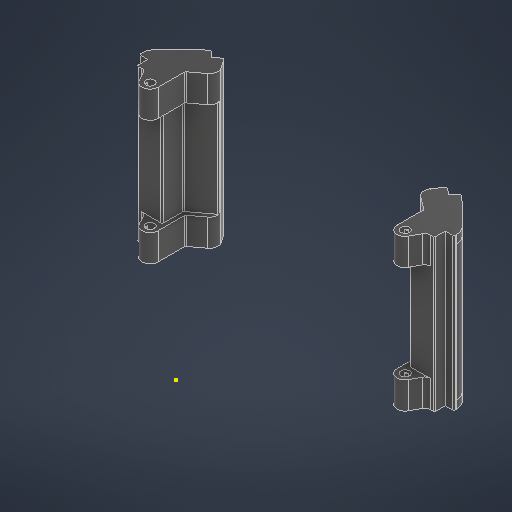
# Autodesk Inventor part: Esquinero Trasero
Saved by Autodesk Inventor 2026.2 (Build 302298000, 298)
## iProperties
Created: 2025-03-12
Part Number: Esquinero Trasero
Material: Generic
Document SubType Name: Modeling
Designer: cdavi
Density: 1 g/cm^3
Appearance: Dark Gray
Author: cdavi
Autodesk Inventor part; units mm, degrees
ref_plane "YZ Plane" through (0, 0, 0) normal (1, 0, 0) x (0, 1, 0)
ref_plane "XZ Plane" through (0, 0, 0) normal (0, 1, 0) x (-1, 0, 0)
ref_plane "XY Plane" through (0, 0, 0) normal (0, 0, 1) x (1, 0, 0)
sketch "Sketch1" plane through (0, 0, 0) normal (0, 1, 0) x (-1, 0, 0)
  line L0 (50.9902, 55) -> (-50.9902, 55)
  line L1 (12, -62.25) -> (-12, -62.25)
  line L2 (-12, -60) -> (12, -60)
  circle A0 centre (0, 0) radius 6
  circle A1 centre (-44.3523, -52.8571) radius 1.5 construction
  circle A2 centre (-41.7906, 34.5) radius 1.5
  circle A3 centre (-20, 51.5) radius 1.5 construction
  circle A4 centre (41.7906, 34.5) radius 1.5
  circle A5 centre (20, 51.5) radius 1.5 construction
  circle A6 centre (44.3523, -52.8571) radius 1.5 construction
  arc A7 (12, -62.25) -> (12, -60) centre (12, -61.125) ccw
  arc A8 (-12, -60) -> (-12, -62.25) centre (-12, -61.125) ccw
  circle A9 centre (0, 0) radius 69 construction
  line L3 (0, 0) -> (0, 55)
  arc A10 (-50.9902, 55) -> (50.9902, 55) centre (0, 0) ccw
  line L4 (0, 0) -> (-75, 0)
  line L5 (0, 0) -> (62.5352, -29.1607) construction
  line L6 (0, 0) -> (69, 0)
  line L7 (0, 0) -> (41.7906, 34.5) construction
  line L8 (50.2232, 23.5) -> (71.2232, 23.5)
  line L9 (71.2232, 23.5) -> (71.2232, -23.5)
  line L10 (71.2232, -23.5) -> (50.2232, -23.5)
  line L11 (50.2232, -23.5) -> (50.2232, 23.5)
  line L12 (50.2232, 23.5) -> (71.2232, -23.5) construction
  line L13 (71.2232, 23.5) -> (50.2232, -23.5) construction
  circle A11 centre (41.8232, -9) radius 1
  circle A12 centre (41.8232, 9) radius 1
  circle A13 centre (16, -12.35) radius 1.5
  circle A14 centre (33.75, -55) radius 1.5
  circle A15 centre (-16, -12.35) radius 1.5
  circle A16 centre (-33.75, -55) radius 1.5
  line L14 (-50.2232, 23.5) -> (-71.2232, 23.5)
  line L15 (-71.2232, 23.5) -> (-71.2232, -23.5)
  line L16 (-71.2232, -23.5) -> (-50.2232, -23.5)
  line L17 (-50.2232, -23.5) -> (-50.2232, 23.5)
  circle A17 centre (-41.8232, -9) radius 1
  circle A18 centre (-41.8232, 9) radius 1
  line L18 (39, -25.5) -> (33, -25.5)
  line L19 (33, -25.5) -> (33, -36.5)
  line L20 (33, -36.5) -> (39, -36.5)
  line L21 (39, -36.5) -> (39, -25.5)
  circle A19 centre (36, -38.5) radius 1
  line L22 (39, -31) -> (33, -31)
  circle A20 centre (36, -23.5) radius 1
  circle A21 centre (40.817, -45.3318) radius 1.5
  circle A22 centre (-41.7906, 34.5) radius 1.5
  circle A23 centre (-40.817, -45.3318) radius 1.5
  line L23 (41.7906, 34.5) -> (41.7906, 39.5)
  line L24 (41.7906, 39.5) -> (63.7554, 39.5) construction
  line L25 (0, 0) -> (44.3523, -52.8571) construction
  line L26 (40.817, -45.3318) -> (0, 0) construction
  line L27 (0, 0) -> (62.5352, 29.1607) construction
  circle A24 centre (10, 6) radius 1.5
  circle A25 centre (-10, 6) radius 1.5
  line L28 (33.2906, 29.5) -> (34.2906, 29.5)
  line L29 (36.2906, 27.5) -> (36.2906, 21.5)
  line L30 (34.2906, 19.5) -> (33.2906, 19.5)
  line L31 (31.2906, 21.5) -> (31.2906, 27.5)
  arc A26 (34.2906, 19.5) -> (36.2906, 21.5) centre (34.2906, 21.5) ccw
  arc A27 (31.2906, 21.5) -> (33.2906, 19.5) centre (33.2906, 21.5) ccw
  arc A28 (33.2906, 29.5) -> (31.2906, 27.5) centre (33.2906, 27.5) ccw
  arc A29 (36.2906, 27.5) -> (34.2906, 29.5) centre (34.2906, 27.5) ccw
  line L32 (0, 0) -> (-41.7906, 34.5) construction
  line L33 (-33.2906, 29.5) -> (-34.2906, 29.5)
  line L34 (-36.2906, 27.5) -> (-36.2906, 21.5)
  line L35 (-34.2906, 19.5) -> (-33.2906, 19.5)
  line L36 (-31.2906, 21.5) -> (-31.2906, 27.5)
  arc A30 (-36.2906, 21.5) -> (-34.2906, 19.5) centre (-34.2906, 21.5) ccw
  arc A31 (-33.2906, 19.5) -> (-31.2906, 21.5) centre (-33.2906, 21.5) ccw
  arc A32 (-31.2906, 27.5) -> (-33.2906, 29.5) centre (-33.2906, 27.5) ccw
  arc A33 (-34.2906, 29.5) -> (-36.2906, 27.5) centre (-34.2906, 27.5) ccw
  circle A34 centre (0, 0) radius 54.1913
  circle A35 centre (0, 0) radius 61 construction
  point P0 (-5.9883, -61.0615)
  point P1 (60.7232, 0)
  point P2 (0, 34.5)
  point P3 (36, -36.5)
  point P4 (50.9902, 55)
  point P5 (0, -6)
  point P6 (31.2906, 29.5)
  point P7 (31.2906, 19.5)
  point P8 (33.7906, 29.5)
  point P9 (-31.2906, 29.5)
  point P10 (-31.2906, 19.5)
  point P11 (-33.7906, 29.5)
  dimension "d12" = 12
  dimension "d287" = 0
  dimension "d398" = 108.3827
  dimension "d0" = 3
  dimension "d1" = 3
  dimension "d15" = 24
  dimension "d16" = 3
  dimension "d62" = 2.25
  dimension "d148" = 3.5
  dimension "d276" = 138
  dimension "d285" = 150
  dimension "d286" = 55
  dimension "d288" = 12
  dimension "d289" = 40
  dimension "d290" = 3.5
  dimension "d291" = 20
  dimension "d293" = 25
  dimension "d300" = 21
  dimension "d301" = 47
  dimension "d304" = 2
  dimension "d305" = 8.4
  dimension "d306" = 9
  dimension "d307" = 3
  dimension "d311" = 16
  dimension "d318" = 33.75
  dimension "d323" = 11
  dimension "d324" = 6
  dimension "d325" = 2
  dimension "d326" = 2
  dimension "d327" = 15
  dimension "d338" = 33
  dimension "d342" = 5
  dimension "d345" = 11
  dimension "d346" = 39.541
  dimension "d348" = 40
  dimension "d350" = 61
  dimension "d351" = 48
  dimension "d352" = 3
  dimension "d353" = 12.35
  dimension "d354" = 55
  dimension "d355" = 25
  dimension "d356" = 60
  dimension "d358" = 71.2232
  dimension "d371" = 3
  dimension "d372" = 10
  dimension "d373" = 6
  dimension "d393" = 5
  dimension "d394" = 10
  dimension "d395" = 5
  dimension "d396" = 2
  dimension "d397" = 8
  constraints: 75 end point, 33 centre point, 30 point on circle, 29 symmetric about line, 11 point on line, 11 tangent, 9 horizontal, 8 coincident, 8 midpoint, 7 parallel, 5 equal radius, 5 perpendicular, 3 vertical, 3 vertical alignment, 1 horizontal alignment, 33 other
  measures "d0" diameter of A4
  measures "d1" diameter of A5
  measures "d15" distance of L1.end L1.start
  measures "d16" diameter of A6
  measures "d62" distance between parallel lines of L1 L2
  measures "d148" distance from line of L0 A5.centre
  measures "d276" diameter of A9
  measures "d285" diameter of A10
  measures "d286" distance from line of L0 point (0, 0)
  measures "d288" horizontal distance of point (0, 0) A7.centre
  measures "d289" distance of A5.centre A3.centre
  measures "d290" distance from line of L0 A3.centre
  measures "d291" distance from line of L3 A5.centre
  measures "d293" angle of L6 L5
  measures "d300" distance of L9.end L10.end
  measures "d301" distance of L10.end L8.start
  measures "d304" diameter of A11
  measures "d305" distance from line of L11 A11.centre
  measures "d306" distance from line of L6 A11.centre
  measures "d307" diameter of A13
  measures "d311" horizontal distance of point (0, 0) A13.centre
  measures "d318" distance from line of L3 A14.centre
  measures "d323" distance of L18.end L19.end
  measures "d324" distance of L18.start L18.end
  measures "d325" distance from line of L10.end L18
  measures "d326" diameter of A19
  measures "d327" distance of A20.centre A19.centre
  measures "d338" distance between parallel lines of L3 L19
  measures "d342" distance of L7.end L23.end
  measures "d345" distance from line of L8 L7.end
  measures "d346" angle of L6 L7
  measures "d348" angle of L3 L25
  measures "d350" distance of L26.start L4.start
  measures "d351" angle of L6 L26
  measures "d352" diameter of A21
  measures "d353" vertical distance of point (0, 0) A13.centre
  measures "d354" distance from line of L6 A14.centre
  measures "d355" angle of L27 L6
  measures "d356" distance between parallel lines of L2 L4
  measures "d358" distance between parallel lines of L3 L15
  measures "d371" diameter of A24
  measures "d372" horizontal distance of A24.centre point (0, 0)
  measures "d373" vertical distance of point (0, 0) A24.centre
  measures "d393" distance between parallel lines of L31 L29
  measures "d394" distance of point (31.291, 19.5) point (31.291, 29.5)
  measures "d395" distance from line of L7.end L28
  measures "d396" radius of A26
  measures "d397" horizontal distance of L7.end point (33.791, 29.5)
extrude "Extrusion1" add sketch "Sketch1" along normal blind 3 contours A10 L8 L11 A34 A4 L3 L0 | L3 A34 A2 L17 L14 A10 L0 | A34 A4 L11 L6 A0 L3 | L3 A0 L4 L17 A34 A2 | A10 L16 L17 A34 L11 L10 | L6 L11 A34 L17 L4 A0
sketch "Sketch3" plane through (0, 3, 0) normal (0, 1, 0) x (1, 0, 0)
  line L0 (3, 0) -> (3, -20)
  circle A0 centre (-10.775, -23.1) radius 1.5
  line L1 (-50.9902, -55) -> (50.9902, -55) projected
  circle A1 centre (16.775, -30.6) radius 1.5
  point P0 (0, 0)
  point P1 (-51.2348, -50)
  dimension "d377" = 20
  dimension "d378" = 3
  dimension "d379" = 3
  dimension "d380" = 13.775
  dimension "d381" = 31.9
  dimension "d383" = 13.775
  dimension "d384" = 3
  dimension "d385" = 24.4
  constraints: 2 centre point, 2 end point, 1 vertical, 1 other
  measures "d377" distance of L0.start L0.end
  measures "d378" distance from line of point (0, 0) L0
  measures "d379" diameter of A0
  measures "d380" distance from line of L0 A0.centre
  measures "d383" distance from line of A1.centre L0
  measures "d384" diameter of A1
fillet "Fillet1" radius 2 1 edges at (71.2232, 1.5, 23.5)
fillet "Fillet2" radius 2 7 edges at (71.2232, 1.5, -23.5) (-71.2232, 1.5, -23.5) (-71.2232, 1.5, 23.5) (-50.2232, 1.5, -23.5) (-50.2232, 1.5, 23.5) (50.2232, 1.5, -23.5) (50.2232, 1.5, 23.5)
hole "Hole1" at (-10.775, 3, 23.1) at (16.775, 3, 30.6) direction (0, -1, 0) diameter 3 end through all
sketch "Sketch4" plane through (0, 3, 0) normal (0, 1, 0) x (1, 0, 0)
  line L0 (-50.2232, 21.5) -> (-50.2232, -21.5) projected
  line L1 (-115.8769, 106.6342) -> (-58.2232, 106.6342)
  line L2 (-58.2232, 106.6342) -> (-58.2232, -77.5521)
  line L3 (-58.2232, -77.5521) -> (-115.8769, -77.5521)
  line L4 (-115.8769, -77.5521) -> (-115.8769, 106.6342)
  line L5 (-50.2232, 0) -> (-58.2232, 0)
  point P0 (0, 0)
  dimension "d403" = 8
  constraints: 10 end point, 2 parallel, 2 perpendicular, 1 horizontal, 1 midpoint, 1 point on line
  measures "d403" distance of L5.start L5.end
extrude "Extrusion3" cut sketch "Sketch4" against normal blind 10
mirror "Mirror1" about plane through (0, 0, 0) normal (1, 0, 0) of "Extrusion3"
fillet "Fillet3" radius 2 4 edges at (-58.2232, 1.5, 23.5) (-58.2232, 1.5, -23.5) (58.2232, 1.5, -23.5) (58.2232, 1.5, 23.5)
sketch "Sketch5" plane through (0, 3, 0) normal (0, 1, 0) x (1, 0, 0)
  point P0 (0, 0)
fillet "Fillet5" [suppressed]
sketch "Sketch6" plane through (0, 3, 0) normal (0, 1, 0) x (1, 0, 0)
  point P0 (0, 0)
sketch "Sketch7" plane through (0, 3, 0) normal (0, 1, 0) x (1, 0, 0)
  arc A0 (58.2232, 47.2764) -> (-58.2232, 47.2764) centre (0, 0) ccw projected
  line L0 (-58.2232, 47.2764) -> (-58.2232, 0)
  line L1 (-58.2232, 0) -> (0, 0)
  constraints: 4 end point, 1 horizontal, 1 vertical
sketch "Sketch8" plane through (0, 3, 0) normal (0, 1, 0) x (1, 0, 0)
  line L0 (58.2232, 47.2764) -> (58.2232, 25.5) projected
  line L1 (58.2232, 47.2764) -> (58.2232, 23)
  point P0 (0, 0)
  constraints: 2 end point, 1 vertical
fillet "Fillet6" radius 5 2 edges at (-58.2232, 1.5, -47.2764) (58.2232, 1.5, -47.2764)
sketch "Sketch9" plane through (0, 3, 0) normal (0, 1, 0) x (1, 0, 0)
  arc A0 (50.9902, -55) -> (58.2232, -47.2764) centre (0, 0) ccw projected
  line L0 (50.9902, -55) -> (58.2232, -55)
  line L1 (58.2232, -55) -> (58.2232, -47.2764)
  circle A1 centre (0, 0) radius 6 projected
  arc A2 (50.9902, -55) -> (58.2232, -47.2764) centre (0, 0) ccw
  constraints: 4 end point, 2 point on circle, 1 centre point, 1 coincident, 1 horizontal, 1 perpendicular
extrude "Extrusion4" add sketch "Sketch9" against normal blind 3 contours A0 L1 L0
mirror "Mirror2" about plane through (0, 0, 0) normal (1, 0, 0) of "Extrusion4"
sketch "Sketch10" plane through (0, 3, 0) normal (0, 1, 0) x (1, 0, 0)
  point P0 (0, 0)
sketch "Sketch11" plane through (0, 3, 0) normal (0, 1, 0) x (1, 0, 0)
  line L0 (-58.2232, -55) -> (58.2232, -55) projected
  line L1 (58.2232, -25.5) -> (58.2232, -55) projected
  line L2 (-58.2232, -55) -> (58.2232, -55)
  line L3 (58.2232, -55) -> (58.2232, -52)
  line L4 (58.2232, -52) -> (-58.2232, -52)
  line L5 (-58.2232, -52) -> (-58.2232, -55)
  point P0 (0, 0)
  dimension "d410" = 3
  constraints: 8 end point, 2 parallel, 1 horizontal, 1 perpendicular, 1 point on line
  measures "d410" distance between parallel lines of L0 L4
extrude "Extrusion5" cut sketch "Sketch11" against normal blind 3
fillet "Fillet7" radius 5 2 edges at (58.2232, 1.5, 52) (-58.2232, 1.5, 52)
sketch "Sketch12" plane through (0, 3, 0) normal (0, 1, 0) x (1, 0, 0)
  arc A0 (-46.2232, 59.0628) -> (-57.0249, 48.7151) centre (0, 0) ccw
  arc A1 (-57.0249, 48.7151) -> (-58.2232, 45.4674) centre (-53.2232, 45.4674) ccw projected
  arc A2 (-57.0249, 48.7151) -> (-58.2232, 45.4674) centre (-53.2232, 45.4674) ccw
  line L0 (-58.2232, 25.5) -> (-58.2232, 45.4674) projected
  line L1 (-58.2232, 40.4674) -> (-58.2232, 45.4674)
  line L2 (-58.2232, 40.4674) -> (-46.2232, 40.4674)
  line L3 (-50.2232, 21.5) -> (-50.2232, -21.5) projected
  line L4 (-46.2232, 40.4674) -> (-46.2232, 59.0628)
  line L5 (76, -57) -> (-111, -57)
  line L6 (-111, -57) -> (-111, 82)
  line L7 (-111, 82) -> (76, 82)
  line L8 (76, 82) -> (76, -57)
  dimension "d414" = 5
  dimension "d415" = 12
  constraints: 14 end point, 4 point on circle, 2 centre point, 2 coincident, 2 parallel, 2 perpendicular, 2 tangent, 1 collinear, 1 horizontal, 1 point on line, 1 vertical
  measures "d414" distance of L0.end L1.start
  measures "d415" distance of L1.start L2.end
extrude "Extrusion6" cut sketch "Sketch12" against normal blind 10
sketch "Sketch14" plane through (0, 3, 0) normal (0, 1, 0) x (1, 0, 0)
  circle A0 centre (-41.2232, 53.4674) radius 1.6
  line L0 (-46.2232, 40.4674) -> (-46.2232, 59.0628) projected
  line L1 (-58.2232, 40.4674) -> (-46.2232, 40.4674) projected
  circle A1 centre (-41.2232, 53.4674) radius 3.05
  line L2 (-41.2232, 56.5174) -> (-46.2232, 56.5174)
  line L3 (-41.2232, 50.4174) -> (-46.2232, 50.4174)
  line L4 (-46.2232, 40.4674) -> (-44.2232, 40.4674)
  line L5 (-44.2232, 40.4674) -> (-44.2232, 50.4174)
  line L6 (-44.2232, 47.4174) -> (-39.3973, 51.0244)
  point P0 (0, 0)
  dimension "d419" = 3.2
  dimension "d420" = 5
  dimension "d421" = 13
  dimension "d422" = 1.45
  dimension "d423" = 2
  dimension "d434" = 3
  constraints: 10 end point, 4 point on line, 3 perpendicular, 3 point on circle, 3 tangent, 2 centre point, 1 coincident, 1 horizontal
  measures "d419" diameter of A0
  measures "d420" distance from line of L0 A0.centre
  measures "d421" distance from line of A0.centre L1
  measures "d422" radial gap between concentric circles of A1 A0
  measures "d423" distance of L0.start L4.end
  measures "d434" distance from line of L3 L6.start
extrude "Extrusion7" add sketch "Sketch14" against normal blind 3
sketch "Sketch15" plane through (0, 3, 0) normal (0, 1, 0) x (1, 0, 0)
  arc A0 (-41.2232, 58.9089) -> (-44, 56.8648) centre (0, 0) ccw
  line L0 (-46.2232, 56.5174) -> (-41.2232, 56.5174) projected
  line L1 (-41.2232, 56.5174) -> (-41.2232, 58.9089)
  line L2 (-46.2232, 56.5174) -> (-41.2232, 56.5174)
  circle A1 centre (-41.2232, 53.4674) radius 1.6 projected
  line L3 (-41.2232, 58.9089) -> (-38.6974, 55.177)
  arc A2 (-39.3973, 51.0244) -> (-41.2232, 56.5174) centre (-41.2232, 53.4674) ccw projected
  line L4 (-41.2232, 56.5174) -> (-41.2232, 56.5174)
  arc A3 (-38.6974, 55.177) -> (-41.2232, 56.5174) centre (-41.2232, 53.4674) ccw
  line L5 (-46.2232, 56.5174) -> (-46.2232, 59.0628) projected
  line L6 (-46.2232, 59.0628) -> (-44, 56.8648)
  line L7 (-46.2232, 59.0628) -> (-46.2232, 56.5174)
  point P0 (-46.2232, 55.0729)
  point P1 (-41.2232, 50.4674)
  point P2 (-45, 56.0768)
  dimension "d427" = 143.8
  dimension "d428" = 0
  dimension "d448" = 2.2232
  constraints: 13 end point, 6 point on circle, 2 centre point, 2 coincident, 2 collinear, 2 perpendicular, 2 tangent, 1 concentric, 1 point on line
  measures "d427" diameter of A0
  measures "d428" distance from line of A1.centre L1
  measures "d448" horizontal distance of L5.end L6.end
extrude "Extrusion8" add sketch "Sketch15" against normal blind 3 contours L1 L0 L5 L6 A0 | L3 A2 L1
sketch "Sketch17" plane through (0, 3, 0) normal (0, 1, 0) x (1, 0, 0)
  line L0 (-58.2232, 45.4674) -> (-58.2232, 40.4674) projected
  line L1 (-58.2232, 40.4674) -> (-58.2232, 45.4674)
  line L2 (-44.2232, 47.4174) -> (-44.2232, 40.4674) projected
  circle A0 centre (-41.2232, 53.4674) radius 1.6 projected
  arc A1 (-41.2232, 58.9089) -> (-44, 56.8648) centre (0, 0) ccw projected
  line L3 (-41.2232, 58.9089) -> (-38.6974, 55.177) projected
  arc A2 (-57.0249, 48.7151) -> (-58.2232, 45.4674) centre (-53.2232, 45.4674) ccw
  arc A3 (-40.5786, 57.9564) -> (-45.7232, 53.9903) centre (0, 0) ccw
  line L4 (-38.6974, 55.177) -> (-41.2232, 58.9089) projected
  line L5 (-40.5786, 57.9564) -> (-41.2232, 58.9089)
  line L6 (-58.2232, 40.4674) -> (-45.7232, 40.4674)
  line L7 (-58.2232, 40.4674) -> (-44.2232, 40.4674) projected
  line L8 (-45.7232, 40.4674) -> (-45.7232, 53.9903)
  arc A4 (-41.2232, 58.9089) -> (-44, 56.8648) centre (0, 0) ccw
  circle A5 centre (0, 0) radius 75
  line L9 (-46.2232, 59.0628) -> (-44, 56.8648) projected
  line L10 (-46.2232, 59.0628) -> (-44, 56.8648)
  point P0 (-58.2232, 45.5014)
  dimension "d492" = 150
  dimension "d435" = 5
  dimension "d439" = 141.5
  dimension "d440" = 1.5
  dimension "d482" = 53.9903
  dimension "d488" = 0
  dimension "d489" = 3
  dimension "d490" = 21.5935
  dimension "d491" = 14
  constraints: 10 end point, 6 point on circle, 3 centre point, 3 collinear, 2 coincident, 2 point on line, 1 concentric, 1 perpendicular, 1 tangent, 5 other
  measures "d435" radius of A2
  measures "d439" diameter of A3
  measures "d440" distance between parallel lines of L2 L8
  measures "d482" vertical distance of point (0, 0) L8.end
  measures "d488" distance from line of point (-41.223, 58.909) L3
  measures "d489" distance from line of point (-41.223, 58.909) L2
  measures "d490" distance from line of point (-58.223, 45.501) L3
  measures "d491" distance from line of point (-58.223, 45.501) L2
extrude "Extrusion9" add sketch "Sketch17" along normal blind 53 contours A2 A5 L9 A1 L3 A3 L8 L6 L0 picked at (-48.3678, 48.9531)
fillet "Fillet11" radius 5 1 edges at (-45.7232, 29.5, -53.9903)
sketch "Sketch18" plane through (0, 56, 0) normal (0, 1, 0) x (1, 0, 0)
  line L0 (-58.2232, 40.4674) -> (-45.7232, 40.4674) projected
  line L1 (-58.2232, 40.4674) -> (-55.0232, 40.4674)
  line L2 (-55.0232, 40.4674) -> (-55.0232, 44.4674)
  line L3 (-55.0232, 44.4674) -> (-58.2232, 44.4674)
  line L4 (-58.2232, 44.4674) -> (-58.2232, 40.4674)
  line L5 (-58.2232, 45.4674) -> (-58.2232, 40.4674) projected
  point P0 (0, 0)
  point P1 (-46.2232, 40.4674)
  dimension "d443" = 3.2
  dimension "d445" = 4
  constraints: 9 end point, 2 parallel, 1 horizontal, 1 perpendicular
  measures "d443" distance of L2.end L3.end
  measures "d445" distance of L1.end L2.end
extrude "Extrusion10" cut sketch "Sketch18" against normal blind 56
sketch "Sketch19" plane through (0, 3, 0) normal (0, 1, 0) x (1, 0, 0)
  circle A0 centre (-41.2232, 53.4674) radius 1.6 projected
  circle A1 centre (-41.2232, 53.4674) radius 1.55
  point P0 (0, 0)
  constraints: 1 centre point, 1 coincident
extrude "Extrusion11" add sketch "Sketch19" against normal blind 3 contours A0 | A1
sketch "Sketch20" plane through (0, 3, 0) normal (0, 1, 0) x (1, 0, 0)
  line L0 (-39.3973, 51.0244) -> (-44.2232, 47.4174) projected
  line L1 (-44.2232, 47.4174) -> (-44.2232, 49.4174)
  line L2 (-44.2232, 47.4174) -> (-44.2232, 40.4674) projected
  arc A0 (-39.3973, 51.0244) -> (-38.6974, 55.177) centre (-41.2232, 53.4674) ccw projected
  line L3 (-44.2232, 49.4174) -> (-38.2062, 53.9146)
  line L4 (-40.5786, 57.9564) -> (-38.6974, 55.177)
  arc A1 (-43.8201, 55.5461) -> (-45.7232, 51.6205) centre (-40.7232, 51.6205) ccw projected
  line L5 (-44.2232, 49.4174) -> (-45.7232, 48.2963)
  line L6 (-45.7232, 51.6205) -> (-45.7232, 48.2963)
  line L7 (-45.7232, 40.4674) -> (-45.7232, 51.6205) projected
  arc A2 (-40.5786, 57.9564) -> (-43.8201, 55.5461) centre (0, 0) ccw projected
  arc A3 (-40.5786, 57.9564) -> (-43.8201, 55.5461) centre (0, 0) ccw
  arc A4 (-38.2062, 53.9146) -> (-38.6974, 55.177) centre (-41.2232, 53.4674) ccw
  dimension "d451" = 2
  constraints: 11 end point, 5 point on circle, 2 centre point, 2 coincident, 2 collinear, 1 parallel, 1 point on line
  measures "d451" distance of L0.end L1.end
extrude "Extrusion12" add sketch "Sketch20" along normal blind 53 contours L3 L5 L6 A1 A2 L4 A0
fillet "Fillet13" radius 0.5 9 edges at (-38.2062, 29.5, -53.9146) (-41.2232, 28, -58.9089) (-46.2232, 1.5, -59.0628) (-46.2232, 29.5, -59.0628) (-45.7232, 29.5, -48.2963) (-44.2232, 1.5, -47.4174) (-45.7232, 29.5, -40.4674) (-55.0232, 28, -40.4674) (-58.2232, 28, -44.4674)
sketch "Sketch21" plane through (0, 3, 0) normal (0, 1, 0) x (1, 0, 0)
  line L0 (-44.2232, 40.4674) -> (-54.5232, 40.4674) projected
  line L1 (-44.2232, 40.4674) -> (-44.2232, 37.4674)
  line L2 (-44.2232, 40.4674) -> (-49.3732, 40.4674)
  circle A0 centre (-47.2232, 37.4674) radius 3
  circle A1 centre (-47.2232, 37.4674) radius 1.6
  line L3 (-44.2232, 40.4674) -> (-52.2232, 40.4674)
  line L4 (-52.2232, 40.4674) -> (-49.8703, 36.0557)
  point P0 (0, 0)
  dimension "d457" = 6
  dimension "d459" = 3.2
  dimension "d460" = 8
  constraints: 8 end point, 3 tangent, 2 centre point, 2 point on circle, 1 coincident, 1 midpoint, 1 point on line, 1 vertical
  measures "d457" diameter of A0
  measures "d459" diameter of A1
  measures "d460" distance from line of L3.end L1
extrude "Extrusion13" add sketch "Sketch21" against normal blind 3
fillet "Fillet14" radius 2 1 edges at (-52.2232, 1.5, -40.4674)
sketch "Sketch22" plane through (0, 0, 0) normal (1, 0, 0) x (0, 1, 0)
  line L0 (0, 0) -> (56, 0)
  line L1 (56, 0) -> (56, -67)
  line L2 (56, -67) -> (0, -67)
  line L3 (0, -67) -> (0, 0)
  line L4 (28, 0) -> (28, -67)
  dimension "d465" = 56
  dimension "d466" = 67
  dimension "d467" = 28
  constraints: 10 end point, 2 midpoint, 2 parallel, 2 perpendicular, 1 horizontal
  measures "d465" distance between parallel lines of L3 L1
  measures "d466" distance of L0.end L1.end
  measures "d467" distance between parallel lines of L1 L4
extrude "Extrusion14" cut sketch "Sketch22" against normal blind 300 contours L0 L1 L2 L4
sketch "Sketch23" plane through (0, 3, 0) normal (0, 1, 0) x (1, 0, 0)
  circle A0 centre (-47.2232, 37.4674) radius 1.6 projected
  circle A1 centre (-47.2232, 37.4674) radius 1.6
  circle A2 centre (-47.2232, 37.4674) radius 3
  line L0 (-53.4232, 40.4674) -> (-54.5232, 40.4674) projected
  line L1 (-53.4232, 40.4674) -> (-46.2232, 40.4674)
  line L2 (-44.2232, 37.4674) -> (-44.2232, 47.1669) projected
  line L3 (-44.2232, 37.4674) -> (-44.2232, 47.1669)
  arc A3 (-44.0226, 47.5674) -> (-44.2232, 47.1669) centre (-43.7232, 47.1669) ccw projected
  line L4 (-44.0226, 47.5674) -> (-39.3973, 51.0244) projected
  line L5 (-44.0226, 47.5674) -> (-39.3973, 51.0244)
  circle A4 centre (-43.7232, 47.1669) radius 0.5
  arc A5 (-38.4602, 53.7248) -> (-38.2765, 54.2543) centre (-38.7596, 54.1253) ccw projected
  circle A6 centre (-38.7596, 54.1253) radius 0.5
  line L6 (-38.4602, 53.7248) -> (-45.5226, 48.4463) projected
  line L7 (-38.4602, 53.7248) -> (-45.5226, 48.4463)
  arc A7 (-45.5226, 48.4463) -> (-45.7232, 48.0458) centre (-45.2232, 48.0458) ccw projected
  circle A8 centre (-45.2232, 48.0458) radius 0.5
  line L8 (-45.7232, 48.0458) -> (-45.7232, 40.9674) projected
  line L9 (-45.7232, 48.0458) -> (-45.7232, 40.9674)
  arc A9 (-46.2232, 40.4674) -> (-45.7232, 40.9674) centre (-46.2232, 40.9674) ccw projected
  circle A10 centre (-46.2232, 40.9674) radius 0.5
  arc A11 (-51.6585, 39.4086) -> (-53.4232, 40.4674) centre (-53.4232, 38.4674) ccw projected
  circle A12 centre (-53.4232, 38.4674) radius 2
  line L10 (-51.6585, 39.4086) -> (-49.8703, 36.0557) projected
  line L11 (-51.6585, 39.4086) -> (-49.8703, 36.0557)
  circle A13 centre (-47.2232, 37.4674) radius 1.3
  line L12 (-47.2232, 37.4674) -> (-49.5232, 37.4674)
  circle A14 centre (-49.5232, 37.4674) radius 1
  circle A15 centre (-47.2232, 37.4674) radius 1.6
  circle A16 centre (-46.0732, 35.4756) radius 1
  circle A17 centre (-47.2232, 37.4674) radius 1.6
  circle A18 centre (-46.0732, 39.4593) radius 1
  arc A19 (-39.3973, 51.0244) -> (-38.2765, 54.2543) centre (-41.2232, 53.4674) ccw projected
  circle A20 centre (-41.2232, 53.4674) radius 3.05
  point P0 (0, 0)
  point P1 (-45.9719, 36.4704)
  point P2 (-46.9855, 35.8852)
  point P3 (-45.9719, 38.4644)
  point P4 (-46.9855, 39.0497)
  point P5 (-48.7124, 36.8822)
  point P6 (-48.7124, 38.0527)
  point P7 (-47.2232, 40.4674)
  dimension "d474" = 3.2
  dimension "d475" = 2.6
  dimension "d476" = 2
  dimension "d479" = 360
  constraints: 14 end point, 10 coincident, 8 centre point, 4 collinear, 2 horizontal, 2 tangent, 1 horizontal alignment, 1 parallel, 1 vertical, 1 vertical alignment, 31 other
  measures "d474" diameter of A1
  measures "d475" diameter of A13
  measures "d476" diameter of A14
extrude "Extrusion15" add sketch "Sketch23" along normal blind 7 contours A0 A18 A2 A16 | A0 A18 A2 | A16 A2 A0 | A0 A14 A2 A18 | A16 A2 A14 A0 | A0 A14 A2 | A18 A2 | A2 L1 A9 L8 A8 L6 A20 L4 A3 L2 A18 | A14 L10 A11 L1 A2 | A2 A14 L10 | A2 L10 A14 | A7 A8 | A20 L6 A5 A19
extrude "Extrusion16" add sketch "Sketch23" along normal blind 6 contours A18 A0 | A0 A16 | A14 L12 A0 | A14 A0 L12
extrude "Extrusion17" add sketch "Sketch23" against normal blind 2 contours A18 A0 | A0 A16 | A14 L12 A0 | A14 A0 L12
mirror "Mirror5" about plane through (0, 28, -67) normal (0, 1, 0)
mirror "Mirror4" about plane through (0, 0, 0) normal (1, 0, 0)
body "Solid1"
